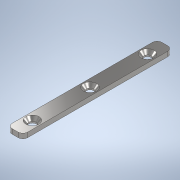
# Autodesk Inventor part: Stencil Clamp - V1
Saved by Autodesk Inventor 2022 (Build 260153000, 153)
## iProperties
Created: 2022-06-23
Part Number: Stencil Clamp - V1
Material: Steel, Mild
Document SubType Name: Modeling
Designer: Caleb
Density: 7.85 g/cm^3
Appearance: Semi-Polished
Author: Caleb
Autodesk Inventor part; units mm, degrees
ref_plane "YZ Plane" through (0, 0, 0) normal (1, 0, 0) x (0, 1, 0)
ref_plane "XZ Plane" through (0, 0, 0) normal (0, 1, 0) x (-1, 0, 0)
ref_plane "XY Plane" through (0, 0, 0) normal (0, 0, 1) x (1, 0, 0)
sketch "Sketch1" plane through (0, 0, 0) normal (0, 1, 0) x (-1, 0, 0)
  line L0 (-2.54, -24.765) -> (2.54, -24.765)
  line L1 (2.54, -24.765) -> (2.54, 24.765)
  line L2 (2.54, 24.765) -> (-2.54, 24.765)
  line L3 (-2.54, 24.765) -> (-2.54, -24.765)
  line L4 (-2.54, -24.765) -> (2.54, 24.765) construction
  line L5 (2.54, -24.765) -> (-2.54, 24.765) construction
  point P0 (0, 0)
  dimension "d0" = 5.08
  dimension "d1" = 49.53
  constraints: 12 end point, 2 midpoint, 2 parallel, 1 horizontal, 1 perpendicular
  measures "d0" distance of L2.end L1.end
  measures "d1" distance of L1.end L0.end
extrude "Extrusion1" add sketch "Sketch1" along normal blind 1.5875
sketch "Sketch2" plane through (0, 1.5875, 0) normal (0, 1, 0) x (1, 0, 0)
  point P0 (0, 0)
  point P1 (0, 0)
  point P2 (0, -19.05)
  point P3 (0, 19.05)
  dimension "d4" = 19.05
  dimension "d5" = 19.05
  constraints: 1 coincident
  measures "d4" distance of point (0, -19.05) point (0, 0)
  measures "d5" distance of point (0, 0) point (0, 19.05)
hole "Hole1" at (0, 1.5875, 0) at (0, 1.5875, 19.05) at (0, 1.5875, -19.05) direction (0, -1, 0) diameter 2.4384 end through all countersink diameter 4.3688 countersink angle 82 clearance for "Flat Head Machine Screw (82)" size "#2" standard "Ansi Unified Screw Threads"
fillet "Fillet1" radius 1.5875 4 edges at (2.54, 0.7937, 24.765) (-2.54, 0.7937, 24.765) (2.54, 0.7937, -24.765) (-2.54, 0.7937, -24.765)
equation "\"d5\" = d4"
body "Solid1"
